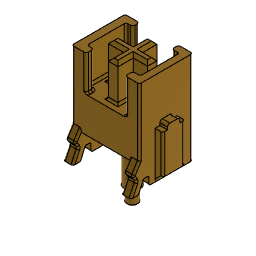
V3_R44 (Autodesk Fusion 360 design; units mm, degrees)
Autodesk Fusion 360 part; units mm, degrees
note: some values were not read from the file. Set by a fixed rule: which face or edge a step refers to.
sketch "Body" plane through (0, 0, 0) normal (0, 0, 1) x (1, 0, 0) in component "Slider"
  line L0 (0, 0) -> (7.1, 0)
  line L1 (7.1, 0) -> (7.1, 5.6)
  line L2 (7.1, 5.6) -> (0, 5.6)
  line L3 (0, 5.6) -> (0, 0)
  dimension "d4" = 7.1
  dimension "d5" = 5.6
  constraint horizontal L0
  constraint vertical L1
  constraint horizontal L2
  constraint vertical L3
  constraint coincident L0.start L3.end
  measures "d4" distance of L0.start L0.end
  measures "d5" distance of L0.start L2.end
extrude "Extrude1" add sketch "Body" along normal blind 6 in component "Slider"
shell "Shell1" thickness 0.44 removed faces 1 at (2.3667, 3.7333, 0) in component "Slider"
sketch "Inner Thick Stem" plane through (0, 0, 5.56) normal (0, 0, -1) x (1, 0, 0) in component "Slider"
  line L0 (0.44, -0.44) -> (0.44, -5.16)
  line L1 (0.44, -5.16) -> (6.66, -5.16)
  line L2 (6.66, -5.16) -> (6.66, -0.44)
  line L3 (6.66, -0.44) -> (0.44, -0.44)
  line L4 (0.44, -0.44) -> (6.66, -5.16) construction
  line L5 (6.66, -0.44) -> (0.44, -5.16) construction
  circle A0 centre (3.55, -2.8) radius 1.6
  dimension "d12" = 3.2
  constraint coincident L0.start L3.end
  constraint coincident L1.end L2.start
  constraint coincident L2.end L3.start
  constraint coincident L0.end L1.start
  constraint midpoint L5 A0.centre
  measures "d12" diameter of A0
extrude "Extrude2" add sketch "Inner Thick Stem" along normal blind 1.4 contours A0 in component "Slider"
sketch "Inner Spring Stem" plane through (0, 0, 4.16) normal (0, 0, -1) x (1, 0, 0) in component "Slider"
  circle A0 centre (3.55, -2.8) radius 1.6
  circle A1 centre (3.55, -2.8) radius 0.825
  dimension "d16" = 1.65
  constraint concentric A0 A1
  measures "d16" diameter of A1
extrude "Extrude3" add sketch "Inner Spring Stem" along normal blind 6.96 contours A1 in component "Slider"
chamfer "Chamfer1" distance 0.775 angle 45 1 edges at (2.0583, 3.3786, 4.16) in component "Slider"
sketch "Cross" plane through (0, 0, 6) normal (0, 0, 1) x (-1, 0, 0) in component "Slider"
  line L0 (0, -5.6) -> (0, 0)
  line L1 (0, 0) -> (-7.1, 0)
  line L2 (-7.1, 0) -> (-7.1, -5.6)
  line L3 (-7.1, -5.6) -> (0, -5.6)
  line L4 (0, -5.6) -> (-7.1, 0) construction
  line L5 (0, 0) -> (-7.1, -5.6) construction
  line L6 (-3.1, -0.75) -> (-4.1, -0.75) construction
  line L7 (-1.5, -2.35) -> (-1.5, -3.35) construction
  line L8 (-4.1, -4.85) -> (-4.1, -3.35)
  line L9 (-4.1, -3.35) -> (-5.6, -3.35)
  line L10 (-5.6, -2.35) -> (-4.1, -2.35)
  line L11 (-4.1, -2.35) -> (-4.1, -0.75)
  line L12 (-4.1, -0.75) -> (-3.1, -0.75)
  line L13 (-3.1, -0.75) -> (-3.1, -2.35)
  line L14 (-3.1, -2.35) -> (-1.5, -2.35)
  line L15 (-1.5, -2.35) -> (-1.5, -3.35)
  line L16 (-1.5, -3.35) -> (-3.1, -3.35)
  line L17 (-3.1, -3.35) -> (-3.1, -4.85)
  line L18 (-3.1, -4.85) -> (-4.1, -4.85)
  line L19 (-5.6, -3.35) -> (-5.6, -2.35)
  dimension "d31" = 1.5
  dimension "d32" = 0.75
  dimension "d35" = 4.1
  dimension "d36" = 4.1
  constraint coincident L0.start L3.end
  constraint coincident L1.end L2.start
  constraint coincident L0.end L1.start
  constraint coincident L2.end L3.start
  constraint horizontal L6
  constraint vertical L7
  constraint perpendicular L8 L18
  constraint perpendicular L10 L19
  measures "d31" distance of L0 L15
  measures "d32" distance of L1 L12
  measures "d35" distance of L7 L19
  measures "d36" distance of L12 L18
extrude "Extrude4" add sketch "Cross" along normal blind 3.75 contours L8 L9 L10 L11 L12 L13 L14 L15 L16 L17 L18 L19 in component "Slider"
chamfer "Chamfer2" distance 0.3 angle 45 12 edges at (2.3, 2.35, 9.75) (1.5, 2.85, 9.75) (2.3, 3.35, 9.75) (3.1, 4.1, 9.75) (3.6, 4.85, 9.75) (4.1, 4.1, 9.75) (4.85, 3.35, 9.75) (5.6, 2.85, 9.75) (4.85, 2.35, 9.75) (4.1, 1.55, 9.75) (3.6, 0.75, 9.75) (3.1, 1.55, 9.75) in component "Slider"
sketch "Wing" plane through (0, 0, 0) normal (-1, 0, 0) x (0, -1, 0) in component "Slider"
  line L0 (-5.6, 0) -> (0, 0)
  line L1 (0, 0) -> (0, 6)
  line L2 (0, 6) -> (-5.6, 6)
  line L3 (-5.6, 6) -> (-5.6, 0)
  line L4 (-5.6, 6) -> (0, 0) construction
  line L5 (0, 6) -> (-5.6, 0) construction
  line L6 (-1.65, 0) -> (-3.95, 0)
  line L7 (-3.95, 0) -> (-3.95, 5.4)
  line L8 (-3.95, 5.4) -> (-1.65, 5.4)
  line L9 (-1.65, 5.4) -> (-1.65, 0)
  line L10 (-1.65, 5.4) -> (-2.15, 5.4)
  line L11 (-2.15, 5.4) -> (-2.15, 4.9)
  line L12 (-2.15, 4.9) -> (-1.65, 4.9)
  line L13 (-1.65, 4.9) -> (-1.65, 5.4)
  line L14 (-3.95, 5.4) -> (-3.45, 5.4)
  line L15 (-3.45, 5.4) -> (-3.45, 4.9)
  line L16 (-3.45, 4.9) -> (-3.95, 4.9)
  line L17 (-3.95, 4.9) -> (-3.95, 5.4)
  point P0 (-2.8, -2.8)
  dimension "d45" = 2.3
  dimension "d46" = 5.4
  dimension "d47" = 1.65
  dimension "d51" = 0.5
  dimension "d52" = 0.5
  dimension "d53" = 0.5
  dimension "d54" = 0.5
  constraint coincident L2.end L3.start
  constraint coincident L0.end L1.start
  constraint coincident L1.end L2.start
  constraint coincident L0.start L3.end
  constraint horizontal L6
  constraint vertical L7
  constraint horizontal L8
  constraint vertical L9
  constraint horizontal L10
  constraint vertical L11
  constraint horizontal L12
  constraint vertical L13
  constraint horizontal L14
  constraint vertical L15
  constraint horizontal L16
  constraint vertical L17
  measures "d45" distance of L6.start L6.end
  measures "d46" distance of L6.start L8.end
  measures "d47" distance of L1 L9
  measures "d51" distance of L8.end L10.end
  measures "d52" distance of L8.end L12.end
  measures "d53" distance of L7.end L14.end
  measures "d54" distance of L7.end L16.end
extrude "Extrude5" add sketch "Wing" along normal blind 0.81 contours L0 L6 L7 L8 L9 L11 L12 L15 L16 in component "Slider"
ref_plane "WorkPlane1" through (3.55, 2.8, 3) normal (-1, 0, 0) x (0, -1, 0) in component "Slider"
mirror "Mirror1" about plane through (3.55, 2.8, 3) normal (-1, 0, 0) of "Extrude5" in component "Slider"
chamfer "Chamfer3" distance 0.81 angle 45 2 edges at (-0.81, 2.8, 0) (7.91, 2.8, 0) in component "Slider"
extrude "Extrude6" add 1 faces at (6.66, 3.5867, 3.7067) along direction (-1, 0, 0) blind 0.56 in component "Slider"
extrude "Extrude7" add 1 faces at (0.44, 3.5867, 1.8533) along direction (1, 0, 0) blind 0.56 in component "Slider"
sketch "Front and Back Cutouts" plane through (0, 0, 0) normal (0, 0, -1) x (1, 0, 0) in component "Slider"
  line L0 (6.1, -5.16) -> (1, -5.16)
  line L1 (1, -5.16) -> (1, -0.44)
  line L2 (1, -0.44) -> (6.1, -0.44)
  line L3 (6.1, -0.44) -> (6.1, -5.16)
  line L4 (7.1, -3.95) -> (7.1, -1.65)
  line L5 (7.1, -1.65) -> (7.1, 0)
  line L6 (7.1, 0) -> (0, 0)
  line L7 (0, 0) -> (0, -1.65)
  line L8 (0, -1.65) -> (0, -3.95)
  line L9 (0, -3.95) -> (0, -5.6)
  line L10 (0, -5.6) -> (7.1, -5.6)
  line L11 (7.1, -5.6) -> (7.1, -3.95)
  line L12 (1, -0.44) -> (6.1, -0.44)
  line L13 (6.1, -0.44) -> (6.1, 0)
  line L14 (6.1, 0) -> (1, 0)
  line L15 (1, 0) -> (1, -0.44)
  line L16 (1, -5.16) -> (6.1, -5.16)
  line L17 (6.1, -5.16) -> (6.1, -5.6)
  line L18 (6.1, -5.6) -> (1, -5.6)
  line L19 (1, -5.6) -> (1, -5.16)
  dimension "d69" = 5.1
  dimension "d88" = 5.1
  constraint horizontal L12
  constraint vertical L13
  constraint horizontal L14
  constraint vertical L15
  constraint coincident L6 L13.end
  constraint coincident L1.end L2.start
  constraint horizontal L16
  constraint vertical L17
  constraint horizontal L18
  constraint vertical L19
  constraint coincident L10 L17.end
  constraint coincident L0.end L1.start
  measures "d69" distance of L1.end L2.end
  measures "d88" distance of L0.end L0.start
extrude "Extrude8" cut sketch "Front and Back Cutouts" against normal blind 2.3 contours L2 L6 L12 L13 L14 L15 in component "Slider"
extrude "Extrude10" cut sketch "Front and Back Cutouts" against normal blind 1 contours L0 L10 L16 L17 L18 L19 in component "Slider"
sketch "Bump" plane through (0, 0, 0) normal (-1, 0, 0) x (0, -1, 0) in component "Slider"
  line L0 (-1.65, 4.9) -> (-1.65, 0)
  line L1 (-1.65, 0) -> (0, 0)
  line L2 (0, 0) -> (0, 6)
  line L3 (0, 6) -> (-5.6, 6)
  line L4 (-5.6, 6) -> (-5.6, 0)
  line L5 (-5.6, 0) -> (-3.95, 0)
  line L6 (-3.95, 0) -> (-3.95, 4.9)
  line L7 (-3.95, 4.9) -> (-3.45, 4.9)
  line L8 (-3.45, 4.9) -> (-3.45, 5.4)
  line L9 (-3.45, 5.4) -> (-2.15, 5.4)
  line L10 (-2.15, 5.4) -> (-2.15, 4.9)
  line L11 (-2.15, 4.9) -> (-1.65, 4.9)
  line L12 (0, 6) -> (0, 2.7) construction
  line L13 (0, 2.7) -> (0.7, 1.6)
  line L14 (0, 0) -> (3.6, 0) construction
  line L15 (0.7, 1.6) -> (0.3, 1)
  line L16 (0, 0) -> (0, -0.3) construction
  line L17 (0, -0.3) -> (0.9, -0.3)
  line L18 (0.9, -0.3) -> (0.3, 1)
  line L19 (0, 0) -> (0, -0.3)
  dimension "d73" = 3.3
  dimension "d74" = 0.7
  dimension "d75" = 1.6
  dimension "d79" = 0.3
  dimension "d82" = 0.6
  dimension "d163" = 0.3
  dimension "d164" = 0.9
  constraint vertical L12
  constraint coincident L2.end L3.start
  constraint coincident L1.end L2.start
  constraint perpendicular L2 L14
  constraint perpendicular L14 L16
  constraint perpendicular L16 L17
  measures "d73" distance of L2.end L12.end
  measures "d74" distance of L2 L13.end
  measures "d75" distance of L13.end L14
  measures "d79" distance of L2 L15.end
  measures "d82" vertical distance of L13.end L15.end
  measures "d163" distance of L1.end L16.end
  measures "d164" distance of L16.end L17.end
extrude "Extrude9" add sketch "Bump" against normal blind 1 contours L2 L13 L15 L17 L18 L19 in component "Slider"
mirror "Mirror2" about plane through (3.55, 2.8, 3) normal (-1, 0, 0) of "Extrude9" in component "Slider"
chamfer "Chamfer4" distance 0.25 angle 45 4 edges at (1, 2.8, 5.56) (3.55, 5.16, 5.56) (6.1, 2.8, 5.56) (3.55, 0.44, 5.56) in component "Slider"
fillet "Fillet1" radius 0.27 4 edges at (0.5, -0.7, 1.6) (6.6, -0.7, 1.6) (0.5, -0.3, 1) (6.6, -0.3, 1) in component "Slider"
fillet "Fillet3" radius 0.25 4 edges at (-0.405, 2.15, 5.4) (-0.405, 3.45, 5.4) (7.505, 3.45, 5.4) (7.505, 2.15, 5.4) in component "Slider"
sketch "Box Top" plane through (0, 0, 6) normal (0, 0, 1) x (-1, 0, 0) in component "Slider"
  line L0 (0, -5.6) -> (0, 0)
  line L1 (0, 0) -> (-7.1, 0)
  line L2 (-7.1, 0) -> (-7.1, -5.6)
  line L3 (-7.1, -5.6) -> (0, -5.6)
  line L4 (-5.6, -3.35) -> (-5.6, -2.35)
  line L5 (-5.6, -2.35) -> (-4.1, -2.35)
  line L6 (-4.1, -2.35) -> (-4.1, -0.75)
  line L7 (-4.1, -0.75) -> (-3.1, -0.75)
  line L8 (-3.1, -0.75) -> (-3.1, -2.35)
  line L9 (-3.1, -2.35) -> (-1.5, -2.35)
  line L10 (-1.5, -2.35) -> (-1.5, -3.35)
  line L11 (-1.5, -3.35) -> (-3.1, -3.35)
  line L12 (-3.1, -3.35) -> (-3.1, -4.85)
  line L13 (-3.1, -4.85) -> (-4.1, -4.85)
  line L14 (-4.1, -4.85) -> (-4.1, -3.35)
  line L15 (-4.1, -3.35) -> (-5.6, -3.35)
  line L16 (-6.4, -4.9) -> (-0.8, -4.9)
  line L17 (-0.8, -4.9) -> (-0.8, -0.8)
  line L18 (-0.8, -0.8) -> (-6.4, -0.8)
  line L19 (-6.4, -0.8) -> (-6.4, -4.9)
  line L20 (-1.5, -2.35) -> (-1.4932, 0) construction
  line L21 (-5.6, -3.35) -> (-5.6062, -5.6) construction
  line L22 (-5.6062, -5.6) -> (-1.4932, -5.6)
  line L23 (-1.4932, -5.6) -> (-1.4932, 0)
  line L24 (-1.4932, 0) -> (-5.6062, 0)
  line L25 (-5.6062, 0) -> (-5.6062, -5.6)
  constraint coincident L9.end L10.start
  constraint coincident L1 L20.end
  constraint coincident L4.start L15.end
  constraint coincident L3 L21.end
  constraint horizontal L22
  constraint vertical L23
  constraint horizontal L24
  constraint vertical L25
  constraint parallel L3 L16
  constraint parallel L0 L17
  constraint parallel L1 L18
  constraint parallel L2 L19
extrude "Extrude14" add sketch "Box Top" along normal blind 3.75 contours L0 L1 L3 L16 L17 L18 L23 | L1 L2 L3 L16 L18 L19 L25 in component "Slider"
fillet "Fillet5" radius 0.25 8 edges at (5.6062, 0, 7.875) (5.6062, 0.8, 7.875) (1.4932, 0, 7.875) (1.4932, 0.8, 7.875) (5.6062, 4.9, 7.875) (5.6062, 5.6, 7.875) (1.4932, 4.9, 7.875) (1.4932, 5.6, 7.875) in component "Slider"
fillet "Fillet6" radius 0.2 4 edges at (0.8, 4.9, 7.875) (0.8, 0.8, 7.875) (6.4, 0.8, 7.875) (6.4, 4.9, 7.875) in component "Slider"
fillet "Fillet7" radius 0.2 34 edges at (1.42, 5.5268, 6) (1.4932, 5.25, 6) (1.42, 4.9732, 6) (1.1216, 4.9, 6) (0.8586, 4.8414, 6) (0.8, 2.85, 6) (0.8586, 0.8586, 6) (1.1216, 0.8, 6) (1.42, 0.7268, 6) (1.4932, 0.4, 6) (1.42, 0.0732, 6) (5.6795, 5.5268, 6) (5.6062, 5.25, 6) (5.6795, 4.9732, 6) (6.0281, 4.9, 6) (6.3414, 4.8414, 6) (6.4, 2.85, 6) (6.3414, 0.8586, 6) (6.0281, 0.8, 6) (5.6795, 0.7268, 6) (5.6062, 0.4, 6) (5.6795, 0.0732, 6) (3.6, 0.75, 6) (3.1, 1.55, 6) (2.3, 2.35, 6) (4.85, 2.35, 6) (4.1, 1.55, 6) (5.6, 2.85, 6) (4.85, 3.35, 6) (4.1, 4.1, 6) (3.6, 4.85, 6) (3.1, 4.1, 6) (2.3, 3.35, 6) (1.5, 2.85, 6) in component "Slider"
chamfer "Chamfer9" distance 0.25 angle 45 1 edges at (2.7808, 3.0983, -2.8) in component "Slider"
fillet "Fillet10" radius 0.2 8 edges at (7.91, 1.65, 2.855) (7.505, 1.65, 0.405) (7.91, 3.95, 2.855) (7.505, 3.95, 0.405) (-0.81, 1.65, 2.855) (-0.405, 1.65, 0.405) (-0.81, 3.95, 2.855) (-0.405, 3.95, 0.405) in component "Slider"
fillet "Fillet11" radius 0.2 24 edges at (0, -0.3028, 2.2242) (0, -0.6478, 1.6006) (0, -0.4931, 1.2897) (0, -0.3393, 0.9969) (0, -0.6317, 0.2814) (0, 0, 6.225) (1, -0.3028, 2.2242) (1, -0.6478, 1.6006) (1, -0.4931, 1.2897) (1, -0.3393, 0.9969) (1, -0.6317, 0.2814) (6.1, -0.3028, 2.2242) (6.1, -0.6478, 1.6006) (6.1, -0.4931, 1.2897) (6.1, -0.3393, 0.9969) (6.1, -0.6317, 0.2814) (7.1, -0.3028, 2.2242) (7.1, -0.6478, 1.6006) (7.1, -0.4931, 1.2897) (7.1, -0.3393, 0.9969) (7.1, -0.6317, 0.2814) (7.1, 0, 6.225) (7.1, 5.6, 4.875) (0, 5.6, 4.875) in component "Slider"
sketch "Sketch2" plane through (0, 0, 0) normal (0, 0, -1) x (1, 0, 0)
  arc A0 (6.9, -5.6) -> (7.1, -5.4) centre (6.9, -5.4) ccw
  line L0 (7.1, -5.4) -> (7.1, -3.75)
  line L1 (7.1, -3.75) -> (7.1, -1.85)
  line L2 (7.1, -1.85) -> (7.1, 0)
  line L3 (7.1, 0) -> (6.1, 0)
  line L4 (6.1, 0) -> (6.1, -5.6)
  line L5 (6.1, -5.6) -> (6.9, -5.6)
  line L6 (7.1, 0) -> (7.1, -1) construction
  circle A1 centre (3.55, -2.8) radius 0.575 construction
  line L7 (3.55, -2.225) -> (3.55, 1.4) construction
  line L8 (7.1, -1) -> (6.1, -1)
  line L9 (6.1, -1) -> (6.1, 0)
  line L10 (6.1, 0) -> (7.1, 0)
  line L11 (7.1, 0) -> (7.1, -1)
  line L12 (0, -1) -> (1, -1)
  line L13 (1, -1) -> (1, 0)
  line L14 (1, 0) -> (0, 0)
  line L15 (0, 0) -> (0, -1)
  dimension "d167" = 1
  constraint coincident L2.end L3.start
  constraint coincident L2 L6.end
  constraint coincident A1 L7.start
  constraint perpendicular L3 L7
  constraint horizontal L8
  constraint vertical L9
  constraint horizontal L10
  constraint vertical L11
  constraint coincident L3.end L4.start
  constraint symmetric L6.end L7 L12.start
  constraint symmetric L7 L8.end L12.end
  constraint symmetric L7 L3.end L13.end
  constraint symmetric L7 L2.end L14.end
  measures "d167" distance of L2.end L6.end
extrude "Extrude17" cut sketch "Sketch2" against normal blind 0.9 contours L2 L3 L4 L8 L9 L10 L11 | L12 L13 L14 L15 in component "Slider"
extrude "Extrude18" cut 2 faces at (0.6667, 0, 0.1) (6.4333, 0, 0.1) along direction (0, -1, 0) blind 0.1 in component "Slider"
draft "Draft2" angle 24 neutral plane through (0, 0, -0.3) pull (0, 0, -1) 2 faces at (0.6667, -0.1, 0.1) (6.4333, -0.1, 0.1) in component "Slider"
fillet "Fillet13" radius 0.15 8 edges at (6.6, 1, 0.9) (6.6, 1, 0) (0.5, 1, 0.9) (0.5, 1, 0) (0.5, 0.4343, 0.9) (6.6, 0.4343, 0.9) (6.6, -0.1, -0.3) (0.5, -0.1, -0.3) in component "Slider"
extrude "Extrude19" add 1 faces at (3.588, 2.625, -2.8) along direction (0, 0, -1) blind 1.35 in component "Slider"
chamfer "Chamfer11" distance 0.125 angle 45 1 edges at (3.0139, 3.0079, -4.15) in component "Slider"
component "Slider" placed x (1, 0, 0) y (0, 1, 0) z (0, 0, 1) at (0, 0, 0)
equation "body_width = 7.1 mm" comment "Slider body width"
equation "body_depth = 5.6 mm" comment "Slider body depth"
equation "body_height = 6 mm" comment "Excluding keycap stem"
equation "d4 = body_width"
equation "d5 = body_depth"
equation "d6 = body_height"
equation "body_walls = 0.44 mm" comment "Recommended max: 0.5mm. Use multiples of extrusion width!"
equation "d9 = body_walls"
equation "spring_thick_dia = 3.2 mm" comment "Outer diameter to grab spring and hold it in place"
equation "spring_thick_height = 1.4 mm" comment "Outer height to grab spring and hold it in place"
equation "d12 = spring_thick_dia"
equation "d13 = spring_thick_height"
equation "spring_stem_dia = 1.65 mm" comment "Inner stem diameter"
equation "d16 = spring_stem_dia"
equation "spring_stem_length = body_height - body_walls - spring_thick_height + leg_downwards_extension_length + 2.5 mm" comment "Inner stem length"
equation "d18 = spring_stem_length"
equation "spring_stem_transition = ( spring_thick_dia - spring_stem_dia ) / 2" comment "Don't edit! Allows for FDM printing without supports"
equation "d21 = spring_stem_transition"
equation "d31 = cross_width_dist"
equation "d32 = cross_depth_dist"
equation "cross_width_dist = ( body_width / 2 ) - ( cross_width / 2 )" comment "Don't edit! Ensures cross is centered"
equation "cross_depth_dist = ( body_depth / 2 ) - ( cross_depth / 2 )" comment "Don't edit! Ensures cross is centered"
equation "d35 = cross_width"
equation "d36 = cross_depth"
equation "cross_width = 4.1 mm" comment "Cross width (for keycap fitment)"
equation "cross_depth = 4.1 mm" comment "Cross depth (for keycap fitment)"
equation "cross_height = 3.75 mm" comment "Height of cross"
equation "d40 = cross_height"
equation "d42 = cross_chamfer"
equation "cross_chamfer = 0.3 mm" comment "Calculated optimal chamfer for the cross"
equation "d45 = wing_width"
equation "d46 = wing_height"
equation "d47 = wing_offset_center"
equation "wing_offset_center = ( body_depth - wing_width ) / 2" comment "Dont edit! Ensures wings are centered"
equation "wing_width = 2.3 mm" comment "Width of guiding wings"
equation "wing_height = 5.4 mm" comment "Height of guiding wings from the bottom"
equation "d51 = wing_cutout"
equation "d52 = wing_cutout"
equation "d53 = wing_cutout"
equation "d54 = wing_cutout"
equation "wing_cutout = 0.5 mm" comment "Box cutout on the top of the wings"
equation "wing_extrusion = 0.81 mm" comment "Amount of how much the wings poke out"
equation "d57 = wing_extrusion"
equation "d59 = -( body_width / 2 )"
equation "d62 = wing_extrusion"
equation "top_chamfer = 0.25 mm" comment "Amount of internal chamfering"
equation "sides_walls = 1 mm - body_walls" comment "Side reinforcement"
equation "d65 = sides_walls"
equation "d67 = sides_walls"
equation "d69 = ( body_width - 2 mm )"
equation "d70 = -front_cutout_height"
equation "front_cutout_height = 2.3 mm" comment "Leg cutout, necessary for Kailh Pro"
equation "d73 = bump_start_fromtop"
equation "d74 = tactile_bump_outside"
equation "d75 = tactile_bump_frombottom"
equation "tactile_bump_frombottom = 1.6 mm" comment "Distance between bump_start_fromtop and where the tactile bump fully extends in Z direction"
equation "tactile_bump_outside = 0.7 mm" comment "How far the tactile bump goes"
equation "d79 = under_bump_outside"
equation "under_bump_dist = 0.6 mm" comment "Distance between section below the bump and the bump itself in Z direction"
equation "under_bump_outside = 0.3 mm" comment "How far the section below the bump goes"
equation "d82 = under_bump_dist"
equation "d88 = ( body_width - 2 mm )"
equation "back_cutout_height = 1 mm" comment "Back cutout, necessary for Kailh Pro"
equation "d90 = -back_cutout_height"
equation "leg_cutout_length = 1 mm" comment "Don't edit! Required cutout on right leg"
equation "leg_cutout_depth = 0.9 mm" comment "Don't edit! Required cutout on right leg"
equation "d104 = top_chamfer"
equation "general_fillet = 0.2 mm" comment "General filleting of the slider, only edit if needed"
equation "d108 = bump_fillet"
equation "bump_fillet = 0.27 mm" comment "Provides smooth transition for tactile bump, only edit if needed"
equation "wing_fillet = wing_cutout / 2" comment "Don't edit! Provides smooth transition for upper portion of the wings"
equation "d114 = wing_fillet"
equation "bump_start_fromtop = 3.3 mm" comment "Where does the bump start (measured from top, excl. cross)"
equation "bump_bottom_outside = 0.9 mm" comment "How much the pre-bump leg extends from the body"
equation "box_walls = 0.8 mm" comment "Wall thickness of the boxed sides"
equation "d134 = cross_height"
equation "d140 = general_fillet"
equation "d144 = general_fillet"
equation "leg_draft = 24 deg" comment "Draft angle of the legs"
equation "d149 = top_chamfer"
equation "over_bump = 1 mm" comment "How long the bump travel expands past the bottom of the stem"
equation "d158 = general_fillet"
equation "d161 = general_fillet"
equation "leg_downwards_extension_length = 0.3 mm" comment "How long the bump travel expands past the bottom of the stem"
equation "d163 = leg_downwards_extension_length"
equation "d164 = bump_bottom_outside"
equation "d167 = leg_cutout_length"
equation "d168 = -leg_cutout_depth"
equation "leg_reduction_depth = 0.1 mm" comment "How much the bump leg is slimmed down by. This value should be determined by trial and error."
equation "d173 = -leg_reduction_depth"
equation "d175 = leg_draft"
equation "d191 = pole_extra_length"
equation "d193 = top_chamfer / 2"
equation "pole_extra_length = 1.35 mm" comment "Smaller diameter extension of the pole"
